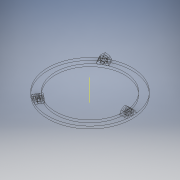
# Autodesk Inventor part: Minimal LED holder
Saved by Autodesk Inventor 2017 (Build 210142000, 142)
## iProperties
Created: 2018-04-03
Part Number: Minimal LED holder
Material: Generic
Document SubType Name: Modeling
Designer: andrew
Density: 1 g/cm^3
Appearance: Default
Author: andrew
Autodesk Inventor part; units mm, degrees
ref_plane "XZ Plane" through (0, 0, 0) normal (0, 1, 0) x (-1, 0, 0)
ref_plane "XY Plane" through (0, 0, 0) normal (0, 0, 1) x (1, 0, 0)
sketch "Sketch1" plane through (0, 0, 0) normal (0, 0, 1) x (1, 0, 0)
  circle A0 centre (0, 0) radius 41
  circle A1 centre (0, 0) radius 50
  dimension "d0" = 82
  dimension "d1" = 100
  constraints: 2 centre point, 2 coincident
  measures "d0" diameter of A0
  measures "d1" diameter of A1
extrude "Extrusion1" add sketch "Sketch1" along normal blind 3
ref_plane "Work Plane1" through (41, 0, 0) normal (1, 0, 0) x (0, 1, 0)
sketch "Sketch2" plane through (41, 0, 0) normal (1, 0, 0) x (0, 1, 0)
  line L0 (0, 5.000565) -> (0, 3)
  line L1 (0, 5.000565) -> (2.000565, 5.000565) construction
  circle A0 centre (0, 5.000565) radius 2 construction
  line L2 (-5.774224, 3.000565) -> (-3.953875, 6.703749)
  line L3 (-2.435898, 3.000565) -> (-5.774224, 3.000565)
  line L4 (2.435941, 3.00059) -> (5.774266, 3.00059)
  line L5 (19.786187, 21.434715) -> (19.786187, 20.434715)
  line L6 (0, 3) -> (0, 3.5)
  line L7 (0, 5.000565) -> (0, 5.250565)
  circle A1 centre (0, 5.250565) radius 1.750565
  line L8 (-2.95, 6.703749) -> (0, 8.406932)
  line L9 (0, 8.406932) -> (2.95, 6.703749)
  line L10 (2.95, 6.703749) -> (2.95, 3.297382)
  line L11 (2.95, 3.297382) -> (0, 1.594199)
  line L12 (0, 1.594199) -> (-2.95, 3.297382)
  line L13 (-2.95, 3.297382) -> (-2.95, 6.703749)
  line L14 (-2.95, 6.703749) -> (-3.953875, 6.703749)
  line L15 (-3.953875, 6.703749) -> (0, 9.500565)
  line L16 (2.95, 6.703749) -> (3.953877, 6.703749)
  line L17 (3.953877, 6.703749) -> (0, 9.500565)
  line L18 (5.774266, 3.00059) -> (3.953877, 6.703749)
  line L19 (-5.774224, 3.000565) -> (-2.435898, 3.000565)
  line L20 (50, 3) -> (-50, 3)
  line L21 (5.774266, 3.00059) -> (2.435941, 3.00059)
  dimension "d36" = 4
  dimension "d37" = 90
  dimension "d46" = 1
  dimension "d50" = 0.5
  dimension "d51" = 0.25
  constraints: 42 end point, 5 coincident, 4 horizontal, 3 point on line, 2 vertical, 1 centre point, 1 collinear, 1 parallel, 1 perpendicular, 1 vertical alignment, 15 other
  measures "d36" diameter of A0
  measures "d37" angle of L0 L1
  measures "d46" distance of L5.start L5.end
  measures "d50" distance of L0.end L6.end
  measures "d51" distance of L7.start L7.end
sketch "Sketch2 outline for Extrusion2" plane through (41, 0, 0) normal (1, 0, 0) x (0, 1, 0)
  line L0 (3.953877, 6.703749) -> (0, 9.500565)
  line L1 (0, 9.500565) -> (-3.953875, 6.703749)
  line L2 (-3.953875, 6.703749) -> (-5.774224, 3.000565)
  line L3 (-5.774224, 3.000565) -> (-2.435898, 3.000565)
  line L4 (-2.435898, 3.000565) -> (0, 1.594199)
  line L5 (0, 1.594199) -> (2.435941, 3.00059)
  line L6 (2.435941, 3.00059) -> (5.774266, 3.00059)
  line L7 (5.774266, 3.00059) -> (3.953877, 6.703749)
  circle A0 centre (0, 5.250565) radius 1.750565
extrude "Extrusion2" add sketch "Sketch2 outline for Extrusion2" along normal blind 3
sketch "Sketch3" plane through (44, 0, 0) normal (1, 0, 0) x (0, 0, -1)
  line L0 (-1.703183, 2.050565) -> (-1.703183, 1.04669)
  circle A0 centre (-5.250565, 0) radius 1.750565
  line L1 (-5.000565, 0) -> (-3, 0)
  circle A1 centre (-5.000565, 0) radius 2 construction
  line L2 (-3.000565, -5.774224) -> (-6.703749, -3.953875)
  line L3 (-3.000565, -2.435898) -> (-3.000565, -5.774224)
  line L4 (-5.000565, 0) -> (-5.000565, 2.000565) construction
  line L5 (-3, 0) -> (-3.5, 0)
  line L6 (-5.000565, 0) -> (-5.250565, 0)
  circle A2 centre (-5.250565, 0) radius 1.750565
  line L7 (-6.703749, -2.95) -> (-8.406932, 0)
  line L8 (-1.594199, 0) -> (-3.297382, -2.95)
  line L9 (-3.297382, -2.95) -> (-6.703749, -2.95)
  line L10 (-6.703749, -2.95) -> (-6.703749, -3.953875)
  line L11 (-6.703749, -3.953875) -> (-9.500565, 0)
  line L12 (-3.000565, -5.774224) -> (-3.000565, -2.435898)
  line L13 (-1.594199, 0) -> (-3.297382, 2.95)
  line L14 (-6.703749, 2.95) -> (-8.406932, 0)
  line L15 (-6.703749, 3.953875) -> (-9.500565, 0)
  line L16 (-3.297382, 2.95) -> (-6.703749, 2.95)
  line L17 (-6.703749, 2.95) -> (-6.703749, 3.953875)
  line L18 (-3.000565, 5.774224) -> (-6.703749, 3.953875)
  line L19 (-3.000565, 2.435898) -> (-3.000565, 5.774224)
  line L20 (-3.000565, 5.774224) -> (-3.000565, 2.435898)
  point P0 (-3.00059, 2.435941)
  constraints: 42 end point, 8 symmetric about line, 5 coincident, 3 point on line, 1 centre point, 1 horizontal alignment, 1 perpendicular, 8 other
extrude "Extrusion3" add sketch "Sketch3" along normal blind 2.8 contours L2 L10 L9 L8 L3 | L18 L19 L13 L16 L17
sketch "Sketch4" plane through (46.8, 0, 0) normal (1, 0, 0) x (0, 0, -1)
  line L0 (-41.626231, 19.374867) -> (-40.626231, 19.374867)
  line L1 (-1.703183, 2.050565) -> (-1.703183, 1.04669) construction
  circle A0 centre (-5.250565, 0) radius 1.750565
  line L2 (-5.000565, 0) -> (-5.000565, 2.000565) construction
  circle A1 centre (-5.250565, 0) radius 1.750565 construction
  line L3 (-5.000565, 0) -> (-5.250565, 0) construction
  circle A2 centre (-5.000565, 0) radius 2 construction
  line L4 (-3, 0) -> (-3.5, 0) construction
  line L5 (-5.000565, 0) -> (-3, 0) construction
  line L6 (-1.594199, 0) -> (-3.297382, -2.95) construction
  line L7 (-6.703749, -2.95) -> (-8.406932, 0) construction
  line L8 (-6.703749, -3.953875) -> (-9.500565, 0) construction
  line L9 (-3.297382, -2.95) -> (-6.703749, -2.95) construction
  line L10 (-6.703749, -2.95) -> (-6.703749, -3.953875) construction
  line L11 (-3.000565, -5.774224) -> (-6.703749, -3.953875) construction
  line L12 (-3.000565, -2.435898) -> (-3.000565, -5.774224) construction
  line L13 (-3.000565, -5.774224) -> (-3.000565, -2.435898) construction
  line L14 (-1.594199, 0) -> (-3.297382, 2.95) construction
  line L15 (-6.703749, 2.95) -> (-8.406932, 0) construction
  line L16 (-6.703749, 3.953875) -> (-9.500565, 0) construction
  line L17 (-3.297382, 2.95) -> (-6.703749, 2.95) construction
  line L18 (-6.703749, 2.95) -> (-6.703749, 3.953875) construction
  line L19 (-3.000565, 2.435898) -> (-3.000565, 5.774224) construction
  line L20 (-3.000565, 5.774224) -> (-3.000565, 2.435898) construction
  line L21 (-3.000565, 5.774224) -> (-6.703749, 3.953875) construction
  line L22 (-3.297382, 2.95) -> (-6.703749, 2.95)
  line L23 (-3.297382, 2.95) -> (-1.594199, 0)
  line L24 (-1.594199, 0) -> (-3.297382, -2.95)
  line L25 (-3.297382, -2.95) -> (-6.703749, -2.95)
  line L26 (-6.703749, -2.95) -> (-8.406932, 0)
  line L27 (-8.406932, 0) -> (-6.703749, 2.95)
  line L28 (-6.703749, 2.95) -> (-3.297382, 2.95)
  point P0 (-3.00059, 2.435941)
  point P1 (-5.000565, 2.95)
  dimension "d48" = 1
  constraints: 56 end point, 8 symmetric about line, 6 coincident, 3 point on line, 2 centre point, 2 midpoint, 1 horizontal, 1 horizontal alignment, 1 perpendicular, 21 other
  measures "d48" distance of L0.start L0.end
extrude "Extrusion4" cut sketch "Sketch4" against normal blind 2.8
sketch "Sketch5" plane through (46.8, 0, 0) normal (1, 0, 0) x (0, 0, -1)
  line L0 (10.262126, 7.665194) -> (12.262691, 7.665194)
  line L1 (12.262101, 10.101135) -> (12.262101, 13.439461)
  circle A0 centre (10.262126, 7.665194) radius 2 construction
  line L2 (12.26214, 1.890995) -> (8.558956, 3.711344)
  line L3 (12.26214, 5.22932) -> (12.26214, 1.890995)
  line L4 (10.262126, 7.665194) -> (10.262126, 9.66576) construction
  line L5 (12.262691, 7.665194) -> (11.762691, 7.665194)
  line L6 (10.262126, 7.665194) -> (10.012126, 7.665194)
  circle A1 centre (10.012126, 7.665194) radius 1.750565
  line L7 (8.558942, 4.715194) -> (6.855759, 7.665194)
  line L8 (6.855759, 7.665194) -> (8.558942, 10.615194)
  line L9 (8.558942, 10.615194) -> (11.965309, 10.615194)
  line L10 (11.965309, 10.615194) -> (13.668492, 7.665194)
  line L11 (13.668492, 7.665194) -> (11.965309, 4.715194)
  line L12 (11.965309, 4.715194) -> (8.558942, 4.715194)
  line L13 (8.558942, 4.715194) -> (8.558956, 3.711344)
  line L14 (8.558956, 3.711344) -> (5.76214, 7.665219)
  line L15 (8.558942, 10.615194) -> (8.558956, 11.619096)
  line L16 (8.558956, 11.619096) -> (5.76214, 7.665219)
  line L17 (12.262101, 13.439461) -> (8.558956, 11.619096)
  line L18 (12.26214, 1.890995) -> (12.26214, 5.22932)
  line L19 (12.262101, 13.439461) -> (12.262101, 10.101135)
  circle A2 centre (-5.250565, 0) radius 1.750565
  line L20 (-5.000565, 0) -> (-3, 0)
  line L21 (-3.00059, 2.435941) -> (-3.00059, 5.774266)
  circle A3 centre (-5.000565, 0) radius 2 construction
  line L22 (-3.000551, -5.774199) -> (-6.703735, -3.953851)
  line L23 (-3.000551, -2.435874) -> (-3.000551, -5.774199)
  line L24 (-5.000565, 0) -> (-5.000565, 2.000565) construction
  line L25 (-3, 0) -> (-3.5, 0)
  line L26 (-5.000565, 0) -> (-5.250565, 0)
  circle A4 centre (-5.250565, 0) radius 1.750565
  line L27 (-6.703749, -2.95) -> (-8.406932, 0)
  line L28 (-8.406932, 0) -> (-6.703749, 2.95)
  line L29 (-6.703749, 2.95) -> (-3.297382, 2.95)
  line L30 (-3.297382, 2.95) -> (-1.594199, 0)
  line L31 (-1.594199, 0) -> (-3.297382, -2.95)
  line L32 (-3.297382, -2.95) -> (-6.703749, -2.95)
  line L33 (-6.703749, -2.95) -> (-6.703735, -3.953851)
  line L34 (-6.703735, -3.953851) -> (-9.500551, 0.000024)
  line L35 (-6.703749, 2.95) -> (-6.703735, 3.953901)
  line L36 (-6.703735, 3.953901) -> (-9.500551, 0.000024)
  line L37 (-3.00059, 5.774266) -> (-6.703735, 3.953901)
  line L38 (-3.000551, -5.774199) -> (-3.000551, -2.435874)
  line L39 (-3.00059, 5.774266) -> (-3.00059, 2.435941)
  constraints: 80 end point, 10 coincident, 6 point on line, 2 centre point, 2 collinear, 2 horizontal alignment, 2 perpendicular, 30 other
extrude "Extrusion5" add sketch "Sketch5" along normal blind 3 contours L30 L29 L35 L37 L21 | L30 L31 L32 L27 L28 L29 | L35 L28 L27 L33 L34 L36 | L23 L22 L33 L32 L31
pattern_circular "Circular Pattern1" count 3 over 360 about axis through (0, 0, 3) along (0, 0, -1) of "Extrusion2", "Extrusion3", "Extrusion4", "Extrusion5"
body "Solid1"
